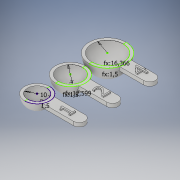
# Autodesk Inventor part: Pigmentlöffel
Saved by Autodesk Inventor 2018.2 (Build 222227000, 227)
## iProperties
Created: 2018-01-23
Part Number: Pigmentlöffel
Material: Generisch
Document SubType Name: Modeling
Designer: JochenAlt
Density: 1 g/cm^3
Appearance: Vorgabe
Author: JochenAlt
Autodesk Inventor part; units mm, degrees
ref_plane "XZ Plane" through (0, 0, 0) normal (0, 1, 0) x (-1, 0, 0)
ref_plane "XY Plane" through (0, 0, 0) normal (0, 0, 1) x (1, 0, 0)
sketch "Skizze1" plane through (0, 0, 0) normal (0, 0, 1) x (1, 0, 0)
  arc A0 (0, -5) -> (0, 5) centre (0, 0) ccw
  arc A1 (0, -6.5) -> (0, 6.5) centre (0, 0) ccw
  line L0 (0, -6.5) -> (0, -5)
  line L1 (0, 5) -> (0, 6.5)
  arc A2 (0, 11.07) -> (0, 23.669) centre (0, 17.3695) ccw
  arc A3 (0, 9.57) -> (0, 25.169) centre (0, 17.3695) ccw
  arc A4 (0, 28.5978) -> (0, 44.9639) centre (0, 36.7809) ccw
  arc A5 (0, 27.0978) -> (0, 46.4639) centre (0, 36.7809) ccw
  line L2 (0, 44.9639) -> (0, 46.4639)
  line L3 (0, 27.0978) -> (0, 28.5978)
  line L4 (0, 9.57) -> (0, 11.07)
  line L5 (0, 23.669) -> (0, 25.169)
  dimension "d0" = 10
  dimension "d8" = 1.5
  dimension "d9" = 12.599
  dimension "d10" = 1.5
  dimension "d11" = 16.3661
  dimension "d12" = 1.5
  constraints: 12 end point, 12 point on circle, 6 centre point, 6 vertical, 4 coincident
  measures "d0" diameter of A0
  measures "d8" radial gap between concentric circles of A1 A0
  measures "d9" diameter of A2
  measures "d10" radial gap between concentric circles of A3 A2
  measures "d11" diameter of A4
  measures "d12" radial gap between concentric circles of A5 A4
revolve "Umdrehung1" add sketch "Skizze1" angle 180 about axis through (0, -6.5, 0) along (0, 1, 0) contours A0 L1 A1 L0
revolve "Umdrehung2" add sketch "Skizze1" angle 180 about axis through (0, 9.57, 0) along (0, 1, 0) contours A2 L5 A3 L4
revolve "Umdrehung3" add sketch "Skizze1" angle 180 about axis through (0, 27.0978, 0) along (0, 1, 0) contours A4 L2 A5 L3
ref_plane "Arbeitsebene1" through (25, 0, 0) normal (1, 0, 0) x (0, 1, 0)
sketch "Skizze3" plane through (25, 0, 0) normal (1, 0, 0) x (0, 1, 0)
  line L0 (-5, 0) -> (5, 0) projected
  line L1 (-3, 0) -> (3, 0)
  line L2 (3, 0) -> (3, -2)
  line L3 (3, -2) -> (-3, -2)
  line L4 (-3, -2) -> (-3, 0)
  line L5 (14.3695, 0) -> (20.3695, 0)
  line L6 (20.3695, 0) -> (20.3695, -2)
  line L7 (20.3695, -2) -> (14.3695, -2)
  line L8 (14.3695, -2) -> (14.3695, 0)
  line L9 (33.7809, 0) -> (39.7809, 0)
  line L10 (39.7809, 0) -> (39.7809, -2)
  line L11 (39.7809, -2) -> (33.7809, -2)
  line L12 (33.7809, -2) -> (33.7809, 0)
  line L13 (25.169, 0) -> (9.57, 0) construction
  line L14 (46.4639, 0) -> (27.0978, 0) construction
  arc A0 (-5, 0) -> (5, 0) centre (0, 0) ccw construction
  line L15 (6.5, 0) -> (-6.5, 0) construction
  line L16 (0, 1.9366) -> (0, -11.6197) construction
  line L17 (-17.0928, 0) -> (57.0567, 0) construction
  line L18 (36.7809, 0) -> (36.7809, -9.6771) construction
  line L19 (17.3695, 0) -> (17.3695, -7.848) construction
  dimension "d16" = 2
  dimension "d17" = 6
  dimension "d21" = 6
  dimension "d22" = 6
  constraints: 28 end point, 6 parallel, 3 coincident, 3 horizontal, 3 perpendicular, 3 point on line, 2 collinear, 2 vertical, 4 other
  measures "d16" distance of the line from the sketch origin of L3
  measures "d17" distance between parallel lines of L2 L4
  measures "d21" distance between parallel lines of L6 L8
  measures "d22" distance between parallel lines of L10 L12
extrude "Extrusion2" add sketch "Skizze3" against normal up to next
fillet "Rundung1" radius 3 6 edges at (25, 3, -1) (25, -3, -1) (25, 14.3695, -1) (25, 20.3695, -1) (25, 33.7809, -1) (25, 39.7809, -1)
sketch "Skizze5" plane through (0, 0, 0) normal (0, 0, 1) x (1, 0, 0)
  line L0 (18.7218, 1.4488) -> (18.7218, -1.527)
  line L1 (18.7218, -1.527) -> (18.099, -1.527)
  line L2 (18.099, -1.527) -> (18.099, -0.4197)
  line L3 (18.099, -0.4197) -> (14.0109, -0.4197)
  line L4 (14.0109, -0.4197) -> (14.0109, -1.527)
  line L5 (14.0109, -1.527) -> (13.4523, -1.527)
  spline S0 degree 2 poles (13.4523, -1.527) (13.4523, -0.8992) (13.0964, -0.306) (12.6021, -0.2665) knots 0 0 0 1 2 2 2
  line L6 (12.6021, -0.2665) -> (12.6021, 0.3663)
  line L7 (12.6021, 0.3663) -> (18.099, 0.3663)
  line L8 (18.099, 0.3663) -> (18.099, 1.4488)
  line L9 (18.099, 1.4488) -> (18.7218, 1.4488)
  line L10 (19.1451, 19.3683) -> (19.1451, 15.6065)
  line L11 (19.1451, 15.6065) -> (18.28, 15.6065)
  spline S1 degree 2 poles (18.28, 15.6065) (17.8994, 16.0118) (17.1925, 16.7336) (16.8119, 17.0796) knots 0 0 0 1 2 2 2
  spline S2 degree 2 poles (16.8119, 17.0796) (16.0457, 17.7766) (15.1262, 18.2858) (14.6368, 18.2858) knots 0 0 0 1 2 2 2
  spline S3 degree 2 poles (14.6368, 18.2858) (14.3798, 18.2858) (13.9942, 18.1276) (13.8706, 17.9842) knots 0 0 0 1 2 2 2
  spline S4 degree 2 poles (13.8706, 17.9842) (13.7471, 17.8409) (13.6235, 17.4652) (13.6235, 17.2378) knots 0 0 0 1 2 2 2
  spline S5 degree 2 poles (13.6235, 17.2378) (13.6235, 17.0203) (13.7322, 16.5754) (13.8163, 16.3727) knots 0 0 0 1 2 2 2
  spline S6 degree 2 poles (13.8163, 16.3727) (13.8855, 16.1997) (14.0832, 15.8784) (14.1524, 15.7795) knots 0 0 0 1 2 2 2
  line L12 (14.1524, 15.7795) -> (14.1524, 15.735)
  line L13 (14.1524, 15.735) -> (13.2824, 15.735)
  spline S7 degree 2 poles (13.2824, 15.735) (13.1588, 15.9871) (12.9166, 16.8918) (12.9166, 17.2971) knots 0 0 0 1 2 2 2
  spline S8 degree 2 poles (12.9166, 17.2971) (12.9166, 18.1523) (13.8212, 19.1162) (14.5924, 19.1162) knots 0 0 0 1 2 2 2
  spline S9 degree 2 poles (14.5924, 19.1162) (14.9532, 19.1162) (15.5563, 18.9482) (15.8133, 18.7999) knots 0 0 0 1 2 2 2
  spline S10 degree 2 poles (15.8133, 18.7999) (16.0803, 18.6516) (16.6043, 18.2215) (16.8564, 17.9842) knots 0 0 0 1 2 2 2
  spline S11 degree 2 poles (16.8564, 17.9842) (17.2765, 17.5986) (18.1762, 16.6545) (18.4382, 16.3727) knots 0 0 0 1 2 2 2
  line L14 (18.4382, 16.3727) -> (18.4382, 19.3683)
  line L15 (18.4382, 19.3683) -> (19.1451, 19.3683)
  line L16 (17.6395, 39.0316) -> (17.6395, 38.3049)
  line L17 (17.6395, 38.3049) -> (19.7355, 38.3049)
  line L18 (19.7355, 38.3049) -> (19.7355, 37.5189)
  line L19 (19.7355, 37.5189) -> (17.6395, 37.5189)
  line L20 (17.6395, 37.5189) -> (17.6395, 34.8249)
  line L21 (17.6395, 34.8249) -> (16.7794, 34.8249)
  line L22 (16.7794, 34.8249) -> (13.6355, 37.5535)
  line L23 (13.6355, 37.5535) -> (13.6355, 38.3049)
  line L24 (13.6355, 38.3049) -> (16.9821, 38.3049)
  line L25 (16.9821, 38.3049) -> (16.9821, 39.0316)
  line L26 (16.9821, 39.0316) -> (17.6395, 39.0316)
  line L27 (16.9821, 37.5189) -> (14.5994, 37.5189)
  line L28 (14.5994, 37.5189) -> (16.9821, 35.4675)
  line L29 (16.9821, 35.4675) -> (16.9821, 37.5189)
  point P0 (0, 0)
  point P1 (12.6021, -2.4514)
  point P2 (12.9166, 15.1616)
  point P3 (13.6355, 34.6617)
  constraints: 3 other
extrude "Extrusion4" add sketch "Skizze5" along normal blind 0.6
equation "\"d9\" = 1.2599 * d0"
equation "\"d10\" = d8"
equation "\"d11\" = 1.299 * d9"
equation "\"d12\" = d10"
equation "\"d21\" = d17"
equation "\"d22\" = d17"
